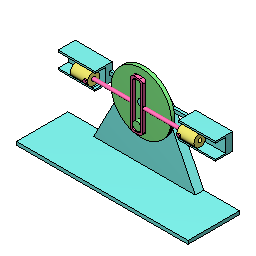
Homework 4 - Scotch Yoke Mechanism v4 (Autodesk Fusion 360 design; units mm, degrees)
Autodesk Fusion 360 part; units mm, degrees
sketch "Holder base" plane through (0, 0, 0) normal (0, 0, 1) x (1, 0, 0) in component "Holder"
  line L0 (100, 30) -> (-100, 30)
  line L1 (-100, 30) -> (-100, -30)
  line L2 (-100, -30) -> (100, -30)
  line L3 (100, -30) -> (100, 30)
  line L4 (100, 30) -> (-100, -30) construction
  line L5 (-100, 30) -> (100, -30) construction
  dimension "d1" = 200
  dimension "d2" = 60
  constraint horizontal L0
  constraint perpendicular L0 L1
  constraint parallel L0 L2
  constraint parallel L1 L3
  constraint coincident L4 origin
  constraint coincident L5 origin
  measures "d1" distance of L1.end L2.end
  measures "d2" distance of L0.end L1.end
extrude "Extrude1" add sketch "Holder base" along normal blind 4 makes body 1 in component "Holder"
sketch "Holder back" plane through (0, 30, 0) normal (0, 1, 0) x (-1, 0, 0) in component "Holder"
  line L0 (-100, 0) -> (100, 0)
  line L1 (100, 0) -> (100, 4)
  line L2 (100, 4) -> (-100, 4)
  line L3 (-100, 4) -> (-100, 0)
  line L4 (-58.4393, 4) -> (-26.9015, 67.8952)
  line L5 (60, 4) -> (26.6392, 68.4138)
  arc A0 (26.6392, 68.4138) -> (-26.9015, 67.8952) centre (0, 54.617) ccw
  line L6 (-0.3188, 84.6153) -> (0.3188, 84.6153)
  constraint coincident L2 L4.start
  constraint tangent L4 A0
  constraint tangent L5 A0
  constraint coincident A0 L6.end
extrude "Extrude2" add sketch "Holder back" against normal blind 10 contours L2 L4 L5 A0 L6 bodies 1 in component "Holder"
sketch "Crank holder" plane through (0, 20, 0) normal (0, -1, 0) x (1, 0, 0) in component "Holder"
  line L0 (-26.6392, 68.4138) -> (-60, 4)
  line L1 (-60, 4) -> (58.4393, 4)
  line L2 (58.4393, 4) -> (26.9015, 67.8952)
  arc A0 (26.9015, 67.8952) -> (-26.6392, 68.4138) centre (0, 54.617) ccw
  circle A1 centre (0, 70.617) radius 4
  dimension "d9" = 8
  measures "d9" diameter of A1
sketch "Crank" plane through (0, 20, 0) normal (0, -1, 0) x (1, 0, 0) in component "Crank"
  circle A0 centre (0, 70.617) radius 35
  dimension "d17" = 70
  measures "d17" diameter of A0
extrude "Extrude1'" add sketch "Crank" along normal blind 4 separate body makes body 2 in component "Crank"
extrude "Extrude2'" cut sketch "Crank holder" along normal blind 5 contours A1 bodies 2 in component "Crank"
extrude "Extrude3" add sketch "Crank holder" along normal blind 5 contours A1 bodies 1 in component "Holder"
move_face "OffsetFaces1" offset -0.3 1 faces at (3.995, 16.6667, 70.4176) on bodies 1 in component "Holder"
sketch "Link slot" plane through (0, 16, 0) normal (0, -1, 0) x (1, 0, 0) in component "Link"
  circle A0 centre (0, 70.617) radius 4
  circle A1 centre (0, 70.617) radius 35
  line L0 (1.5, 97) -> (-1.5, 97)
  line L1 (-5, 93.5) -> (-5, 47.7339)
  line L2 (-1.5, 44.2339) -> (1.5, 44.2339)
  line L3 (5, 47.7339) -> (5, 93.5)
  line L4 (5, 97) -> (-5, 44.2339) construction
  line L5 (-5, 97) -> (5, 44.2339) construction
  line L6 (7, 45.7339) -> (7, 95.5)
  line L7 (3.5, 99) -> (-3.5, 99)
  line L8 (-7, 95.5) -> (-7, 45.7339)
  line L9 (-3.5, 42.2339) -> (3.5, 42.2339)
  arc A2 (-3.5, 99) -> (-7, 95.5) centre (-3.5, 95.5) ccw
  arc A3 (7, 95.5) -> (3.5, 99) centre (3.5, 95.5) ccw
  arc A4 (3.5, 42.2339) -> (7, 45.7339) centre (3.5, 45.7339) ccw
  arc A5 (-7, 45.7339) -> (-3.5, 42.2339) centre (-3.5, 45.7339) ccw
  arc A6 (-1.5, 97) -> (-5, 93.5) centre (-1.5, 93.5) ccw
  arc A7 (5, 93.5) -> (1.5, 97) centre (1.5, 93.5) ccw
  arc A8 (1.5, 44.2339) -> (5, 47.7339) centre (1.5, 47.7339) ccw
  arc A9 (-5, 47.7339) -> (-1.5, 44.2339) centre (-1.5, 47.7339) ccw
  point P0 (0, 70.617)
  dimension "d33" = 3.5
  dimension "d34" = 3.5
  dimension "d35" = 3.5
  constraint horizontal L0
  constraint perpendicular L0 L1
  constraint parallel L0 L2
  constraint parallel L1 L3
  constraint coincident L4 P0
  constraint coincident L5 P0
  constraint coincident P0 A0.centre
  constraint parallel L3 L6
  constraint parallel L0 L7
  constraint parallel L1 L8
  constraint parallel L2 L9
  constraint tangent L7 A2
  constraint tangent L8 A2
  constraint tangent L6 A3
  constraint tangent L7 A3
  constraint tangent L6 A4
  constraint tangent L9 A4
  constraint equal A3 A4
  constraint tangent L8 A5
  constraint tangent L9 A5
  constraint equal A3 A5
  constraint coincident L5.start L1
  constraint coincident L5.start L0
  constraint tangent L1 A6
  constraint tangent L0 A6
  constraint coincident L4.start L0
  constraint coincident L4.start L3
  constraint tangent L0 A7
  constraint tangent L3 A7
  constraint equal A6 A7
  constraint coincident L5.end L3
  constraint coincident L5.end L2
  constraint tangent L3 A8
  constraint tangent L2 A8
  constraint equal A6 A8
  constraint coincident L4.end L2
  constraint coincident L4.end L1
  constraint tangent L2 A9
  constraint tangent L1 A9
  constraint equal A6 A9
  measures "d33" radius of A2
  measures "d34" radius of A3
  measures "d35" radius of A6
extrude "Extrude3'" add sketch "Link slot" along normal blind 4 separate body contours L6 L7 L8 L9 A2 A3 A4 A5 makes body 3 in component "Link"
sketch "Crank pin" plane through (0, 10.7343, 0) normal (0, -1, 0) x (1, 0, 0) in component "Crank"
  arc A0 (-5, 47.5106) -> (-1.5, 44.0106) centre (-1.5, 47.5106) ccw
  line L0 (-5, 47.5106) -> (-5, 93.2766)
  arc A1 (-1.5, 96.7766) -> (-5, 93.2766) centre (-1.5, 93.2766) ccw
  line L1 (-1.5, 96.7766) -> (1.5, 96.7766)
  arc A2 (5, 93.2766) -> (1.5, 96.7766) centre (1.5, 93.2766) ccw
  line L2 (5, 93.2766) -> (5, 47.5106)
  arc A3 (1.5, 44.0106) -> (5, 47.5106) centre (1.5, 47.5106) ccw
  line L3 (1.5, 44.0106) -> (-1.5, 44.0106)
  arc A4 (-7, 45.5106) -> (-3.5, 42.0106) centre (-3.5, 45.5106) ccw
  line L4 (-3.5, 42.0106) -> (3.5, 42.0106)
  arc A5 (3.5, 42.0106) -> (7, 45.5106) centre (3.5, 45.5106) ccw
  line L5 (7, 45.5106) -> (7, 95.2766)
  arc A6 (7, 95.2766) -> (3.5, 98.7766) centre (3.5, 95.2766) ccw
  line L6 (3.5, 98.7766) -> (-3.5, 98.7766)
  arc A7 (-3.5, 98.7766) -> (-7, 95.2766) centre (-3.5, 95.2766) ccw
  line L7 (-7, 95.2766) -> (-7, 45.5106)
  circle A8 centre (0, 50) radius 4.75
  dimension "d39" = 9.5
  measures "d39" diameter of A8
extrude "Extrude3''" add sketch "Crank pin" against normal blind 6 contours A8 bodies 2 in component "Crank"
sketch "link arm right" plane through (7, 0, 0) normal (1, 0, 0) x (0, 1, 0) in component "Link"
  line L0 (16, 45.7339) -> (16, 95.5)
  line L1 (16, 95.5) -> (12, 95.5)
  line L2 (12, 95.5) -> (12, 45.7339)
  line L3 (12, 45.7339) -> (16, 45.7339)
  line L4 (12, 45.7339) -> (16, 95.5) construction
  line L5 (12, 95.5) -> (16, 45.7339) construction
  circle A0 centre (14, 70.617) radius 2
  dimension "d42" = 4
  constraint coincident L2.end L3.start
  constraint coincident L0.end L1.start
  constraint coincident L1.end L2.start
  constraint coincident L0.start L3.end
  constraint midpoint L4 A0.centre
  measures "d42" diameter of A0
extrude "Extrude4" add sketch "link arm right" along normal blind 50 contours A0 bodies 3 in component "Link"
sketch "link arm left" plane through (-7, 0, 0) normal (-1, 0, 0) x (0, -1, 0) in component "Link"
  line L0 (-16, 95.5) -> (-16, 45.7339)
  line L1 (-16, 45.7339) -> (-12, 45.7339)
  line L2 (-12, 45.7339) -> (-12, 95.5)
  line L3 (-12, 95.5) -> (-16, 95.5)
  line L4 (-16, 95.5) -> (-12, 45.7339) construction
  line L5 (-16, 45.7339) -> (-12, 95.5) construction
  circle A0 centre (-14, 70.617) radius 2
  dimension "d45" = 4
  constraint coincident L0.start L3.end
  constraint coincident L1.end L2.start
  constraint coincident L0.end L1.start
  constraint coincident L2.end L3.start
  constraint midpoint L4 A0.centre
  measures "d45" diameter of A0
extrude "Extrude5" add sketch "link arm left" along normal blind 50 contours A0 bodies 3 in component "Link"
sketch "Slider" plane through (57, 0, 0) normal (1, 0, 0) x (0, 1, 0) in component "Sliders"
  circle A0 centre (12.7343, 70.3936) radius 2
  circle A1 centre (12.7343, 70.3936) radius 7
  dimension "d48" = 5
extrude "Extrude1''" add sketch "Slider" along normal blind 20 separate body makes body 4 in component "Sliders"
move_face "OffsetFaces1'" offset -0.3 1 faces at (70.3333, 14.6136, 71.0776) on bodies 4 in component "Sliders"
move_body "Move1" bodies 4 to x (1, 0, 0) y (0, 1, 0) z (0, 0, 1) at (-7.2875, 0, 0) in component "Sliders"
copy_body "CopyPasteBodies1" bodies 4 makes body 5 in component "Sliders"
move_body "Move2" bodies 5 to x (1, 0, 0) y (0, 1, 0) z (0, 0, 1) at (-119.9997, 0, 0.202) in component "Sliders"
move_body "Move3" bodies 5 to x (1, 0, 0) y (0, 1, 0) z (0, 0, 1) at (5, 0, 0) in component "Sliders"
move_body "Move4" bodies 4 to x (1, 0, 0) y (0, 1, 0) z (0, 0, 1) at (15, 0, 0) in component "Sliders"
move_body "Move5" bodies 4 to x (1, 0, 0) y (0, 1, 0) z (0, 0, 1) at (-5, 0, 0) in component "Sliders"
sketch "link-slider pin right" plane through (0, 12, 0) normal (0, -1, 0) x (1, 0, 0) in component "Link"
  arc A0 (-5, 47.7339) -> (-1.5, 44.2339) centre (-1.5, 47.7339) ccw
  line L0 (-5, 47.7339) -> (-5, 93.5)
  arc A1 (-1.5, 97) -> (-5, 93.5) centre (-1.5, 93.5) ccw
  line L1 (-1.5, 97) -> (1.5, 97)
  arc A2 (5, 93.5) -> (1.5, 97) centre (1.5, 93.5) ccw
  line L2 (5, 93.5) -> (5, 47.7339)
  arc A3 (1.5, 44.2339) -> (5, 47.7339) centre (1.5, 47.7339) ccw
  line L3 (1.5, 44.2339) -> (-1.5, 44.2339)
  arc A4 (-7, 45.7339) -> (-3.5, 42.2339) centre (-3.5, 45.7339) ccw
  line L4 (-3.5, 42.2339) -> (3.5, 42.2339)
  arc A5 (3.5, 42.2339) -> (7, 45.7339) centre (3.5, 45.7339) ccw
  line L5 (7, 45.7339) -> (7, 70.617)
  line L6 (7, 70.617) -> (7, 95.5)
  arc A6 (7, 95.5) -> (3.5, 99) centre (3.5, 95.5) ccw
  line L7 (3.5, 99) -> (-3.5, 99)
  arc A7 (-3.5, 99) -> (-7, 95.5) centre (-3.5, 95.5) ccw
  line L8 (-7, 95.5) -> (-7, 70.617)
  line L9 (-7, 70.617) -> (-7, 45.7339)
  line L10 (54.7306, 72.4086) -> (54.7315, 72.4086)
  line L11 (54.7315, 68.4086) -> (54.7306, 68.4086)
  circle A8 centre (54.7311, 70.4086) radius 2
  dimension "d52" = 4
  constraint horizontal L10
  constraint horizontal L11
  constraint coincident A8 L10.start
  constraint coincident A8 L10.end
  constraint coincident A8 L11.start
  constraint coincident A8 L11.end
  measures "d52" diameter of A8
extrude "Extrude6" add sketch "link-slider pin right" along normal blind 6 contours A8 bodies 3 in component "Link"
extrude "Extrude2''" cut sketch "link-slider pin right" along normal blind 11 contours A8 sketch seen with x (1, 0, 0) y (0, 1, 0) z (0, 0, 1) at (7.7125, -1.2657, -0.2234) bodies 4 in component "Sliders"
sketch "link-slider pin left" plane through (0, 12, 0) normal (0, -1, 0) x (1, 0, 0) in component "Link"
  circle A0 centre (-54.7, 70.6) radius 2
  dimension "d57" = 4
  measures "d57" diameter of A0
extrude "Extrude7" add sketch "link-slider pin left" along normal blind 6 separate body makes body 6 in component "Link"
move_body "Move6" bodies 5 to x (1, 0, 0) y (0, 1, 0) z (0, 0, 1) at (0.9173, 0, 0) in component "Sliders"
extrude "Extrude3'''" cut sketch "link-slider pin left" along normal blind 26 sketch seen with x (1, 0, 0) y (0, 1, 0) z (0, 0, 1) at (7.7125, -1.2657, -0.2234) bodies 5 in component "Sliders"
move_face "OffsetFaces2" offset -0.3 1 faces at (-48.5729, 9.0508, 71.5959) on bodies 5 in component "Sliders"
sketch "holder arms" plane through (0, 30, 0) normal (0, 1, 0) x (-1, 0, 0) in component "Holder"
  line L0 (-100, 0) -> (100, 0)
  line L1 (100, 0) -> (100, 4)
  line L2 (100, 4) -> (60, 4)
  line L3 (60, 4) -> (26.6392, 68.4138)
  arc A0 (26.6392, 68.4138) -> (-26.9015, 67.8952) centre (0, 54.617) ccw
  line L4 (-26.9015, 67.8952) -> (-58.4393, 4)
  line L5 (-58.4393, 4) -> (-100, 4)
  line L6 (-100, 4) -> (-100, 0)
  line L7 (-26.9015, 67.8952) -> (-24.5616, 71.8427)
  line L8 (-49, 60) -> (-91.9096, 59.9911)
  line L9 (-91.9096, 59.9911) -> (-91.9096, 79.9911)
  line L10 (-91.9096, 79.9911) -> (-49, 80)
  line L11 (-49, 80) -> (-49, 60)
  line L12 (-24.5616, 71.8427) -> (-49, 71.8427)
  line L13 (-26.9015, 67.8952) -> (-49, 67.8952)
  line L14 (-0.2906, 84.6156) -> (0, 0)
  line L15 (24.0676, 72.0097) -> (48.5054, 72.1776)
  line L16 (26.4345, 68.0784) -> (48.5325, 68.2301)
  line L17 (26.4345, 68.0784) -> (24.0676, 72.0097)
  line L18 (48.4494, 80.3346) -> (48.5868, 60.3351)
  line L19 (91.358, 80.6204) -> (48.4494, 80.3346)
  line L20 (91.4954, 60.6209) -> (91.358, 80.6204)
  line L21 (48.5868, 60.3351) -> (91.4954, 60.6209)
  constraint coincident A0 L7.end
  constraint coincident A0.end L4.start
  constraint coincident L11 L12.end
  constraint perpendicular L11 L12
  constraint coincident L11 L13.end
  constraint perpendicular L11 L13
  constraint midpoint A0 L14.start
  constraint coincident L14.end origin
  constraint symmetric L7.end L14 L15.start
  constraint symmetric A0.end L14 L16.start
  constraint symmetric L8.start L14 L18.end
  constraint symmetric L8.end L14 L20.start
  constraint symmetric L9.end L14 L19.start
  constraint symmetric L10.end L14 L18.start
  constraint symmetric L12.end L14 L15.end
  constraint symmetric L13.end L14 L16.end
extrude "Extrude4'" add sketch "holder arms" against normal blind 3 contours A0 L11 L12 L13 | L3 A0 L15 L16 L18 bodies 1 in component "Holder"
extrude "Extrude5'" add sketch "holder arms" against normal blind 20 contours L8 L9 L10 L11 | L18 L19 L20 L21 bodies 1 in component "Holder"
sketch "holder arms holes" plane through (0, 10, 0) normal (0, -1, 0) x (1, 0, 0) in component "Holder"
  line L0 (91.9096, 79.9911) -> (49, 80)
  line L1 (49, 80) -> (49, 60)
  line L2 (49, 60) -> (91.9096, 59.9911)
  line L3 (91.9096, 59.9911) -> (91.9096, 79.9911)
  line L4 (52, 61.7543) -> (49, 61.7543)
  line L5 (92.1866, 61.746) -> (52, 61.7543)
  line L6 (92.1866, 77.9916) -> (92.1866, 61.746)
  line L7 (52, 78) -> (92.1866, 77.9916)
  line L8 (52, 78) -> (49, 78)
  line L9 (0.2906, 84.6156) -> (0, 0)
  line L10 (-91.6488, 78.6229) -> (-91.7604, 62.3776)
  line L11 (-91.7604, 62.3776) -> (-51.5746, 62.11)
  line L12 (-51.4631, 78.3553) -> (-91.6488, 78.6229)
  line L13 (-51.4631, 78.3553) -> (-48.4631, 78.3347)
  line L14 (-51.5746, 62.11) -> (-48.5747, 62.0894)
  line L15 (-48.4631, 78.3347) -> (-48.5747, 62.0894)
  constraint symmetric L4.start L9 L11.end
  constraint symmetric L4.end L9 L14.end
  constraint symmetric L5.start L9 L10.end
  constraint symmetric L6.start L9 L10.start
  constraint symmetric L7.start L9 L12.start
  constraint symmetric L8.end L9 L13.end
  constraint perpendicular L14 L15
extrude "Extrude6'" cut sketch "holder arms holes" against normal blind 12 contours L3 L5 L6 L7 | L1 L3 L4 L5 L7 L8 | L10 L11 L12 L13 L14 L15 bodies 1 in component "Holder"
extrude "Extrude8" [no effect] in component "Link"
extrude "Extrude4''" [no effect] in component "Sliders"
combine "Combine1" operation add target body 6 tool bodies 3 in component "Link"
component "Holder" placed x (1, 0, 0) y (0, 1, 0) z (0, 0, 1) at (0.0103, 0.5355, 0.5252)
component "Crank" placed x (1, 0, 0) y (0, 1, 0) z (0, 0, 1) at (0, 0, 0)
component "Link" placed x (1, 0, 0) y (0, 1, 0) z (0, 0, 1) at (0, -1.2657, -0.2234)
component "Sliders" placed x (1, 0, 0) y (0, 1, 0) z (0, 0, 1) at (-7.7125, 0, 0)
named bodies: "Holder", "Crank", "Link", "Slider right", "Slider left"
